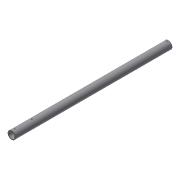
# Autodesk Inventor part: Wind Turbine Pole
Saved by Autodesk Inventor 2015 SP1 (Build 190203100, 203)
## iProperties
Created: 2015-08-24
Part Number: Wind Turbine Pole
Material: 一般
Document SubType Name: Modeling
Designer: nobuhiro
Density: 1 g/cm^3
Appearance: 既定
Author: nobuhiro
Autodesk Inventor part; units mm, degrees
ref_plane "YZ Plane" through (0, 0, 0) normal (1, 0, 0) x (0, 1, 0)
ref_plane "XZ Plane" through (0, 0, 0) normal (0, 1, 0) x (-1, 0, 0)
ref_plane "XY Plane" through (0, 0, 0) normal (0, 0, 1) x (1, 0, 0)
sketch "スケッチ1" plane through (0, 0, 0) normal (0, 0, 1) x (1, 0, 0)
  line L0 (47.5, 0) -> (57, 0)
  line L1 (57, 0) -> (57, 2290)
  line L2 (57, 2290) -> (47.5, 2290)
  line L3 (47.5, 2290) -> (47.5, 0)
  line L4 (0, 0) -> (0, 2264.8884) construction
  dimension "d0" = 2290
  dimension "d1" = 47.5
  dimension "d2" = 57
  constraints: 10 end point, 2 parallel, 1 horizontal, 1 perpendicular, 1 vertical
  measures "d0" distance of L0.end L1.end
  measures "d1" distance between parallel lines of L3 L4
  measures "d2" distance between parallel lines of L4 L1
revolve "回転1" add sketch "スケッチ1" angle 360 about axis through (0, 0, 0) along (0, 1, 0)
sketch "スケッチ2" plane through (0, 0, 0) normal (0, 0, 1) x (1, 0, 0)
  circle A0 centre (0, 45) radius 6
  circle A1 centre (0, 295) radius 6
  circle A2 centre (0, 2270) radius 6
  line L0 (-47.5, 2290) -> (47.5, 2290) projected
  point P0 (0, 0)
  dimension "d6" = 45
  dimension "d7" = 295
  dimension "d8" = 12
  dimension "d15" = 20
  constraints: 3 centre point, 3 vertical alignment, 2 equal radius
  measures "d6" distance of A0.centre point (0, 0)
  measures "d7" distance of point (0, 0) A1.centre
  measures "d8" diameter of A0
  measures "d15" distance from line of L0 A2.centre
extrude "押し出し1" cut sketch "スケッチ2" along normal through all both and the other way through all
sketch "スケッチ3" plane through (0, 0, 0) normal (1, 0, 0) x (0, 1, 0)
  circle A0 centre (175, 0) radius 6
  point P0 (0, 0)
  dimension "d11" = 12
  dimension "d12" = 175
  constraints: 1 centre point, 1 horizontal alignment
  measures "d11" diameter of A0
  measures "d12" distance of point (0, 0) A0.centre
extrude "押し出し2" cut sketch "スケッチ3" along normal through all both and the other way through all
sketch "スケッチ4" plane through (0, 0, 0) normal (1, 0, 0) x (0, 1, 0)
  line L0 (2290, -57) -> (0, -57) projected
  line L1 (2290, 57) -> (2290, -57) projected
  line L2 (0, 57) -> (0, -57) projected
  line L3 (985, -57) -> (1015, -57)
  line L4 (1015, -57) -> (1015, -57.1)
  line L5 (1015, -57.1) -> (985, -57.1)
  line L6 (985, -57.1) -> (985, -57)
  line L7 (1985, -57) -> (2015, -57)
  line L8 (2015, -57) -> (2015, -57.1)
  line L9 (2015, -57.1) -> (1985, -57.1)
  line L10 (1985, -57.1) -> (1985, -57)
  line L11 (1000, -57.1) -> (1000, -57) construction
  line L12 (2000, -57.1) -> (2000, -57) construction
  line L13 (0, 0) -> (2290, 0) construction
  dimension "d16" = 0.1
  dimension "d17" = 30
  dimension "d18" = 1000
  dimension "d19" = 2000
  constraints: 22 end point, 5 midpoint, 4 parallel, 2 equal length, 2 horizontal, 2 perpendicular, 2 point on line
  measures "d16" distance of L5.end L3.start
  measures "d17" distance of L4.end L5.end
  measures "d18" distance between parallel lines of L2 L11
  measures "d19" distance between parallel lines of L12 L2
revolve "回転2" add sketch "スケッチ4" angle 360 about axis through (0, 0, 0) along (0, 1, 0)
